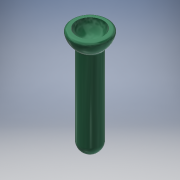
# Autodesk Inventor part: Component 4 (Pound)
Saved by Autodesk Inventor 2018 (Build 220112000, 112)
## iProperties
Created: 2023-03-14
Part Number: Component 4 (Pound)
Material: Generic
Document SubType Name: Modeling
Designer: Habib Mohamed
Density: 1 g/cm^3
Appearance: Olive Green
Author: Habib Mohamed
Autodesk Inventor part; units mm, degrees
ref_plane "YZ Plane" through (0, 0, 0) normal (1, 0, 0) x (0, 1, 0)
ref_plane "XZ Plane" through (0, 0, 0) normal (0, 1, 0) x (-1, 0, 0)
ref_plane "XY Plane" through (0, 0, 0) normal (0, 0, 1) x (1, 0, 0)
sketch "Sketch1" plane through (0, 0, 0) normal (1, 0, 0) x (0, 1, 0)
  line L0 (0, 0) -> (20, 0) construction
  arc A0 (20, 2.5) -> (17.5, 0) centre (20, 0) ccw
  arc A1 (19.4167, 3.451) -> (17.2678, 2.1875) centre (20, 0) ccw
  line L1 (2, 2) -> (16.8775, 2)
  line L2 (2, 2) -> (2, -2.5) construction
  arc A2 (2, 2) -> (0.0157, 0.25) centre (2, 0) ccw
  line L3 (0.25, 0) -> (0.0157, 0.25)
  line L4 (20, 0) -> (20, 2.958)
  line L5 (17.5, 0) -> (0.25, 0)
  arc A3 (20, 2.958) -> (19.4167, 3.451) centre (19.5, 2.958) ccw
  arc A4 (16.8775, 2) -> (17.2678, 2.1875) centre (16.8775, 2.5) ccw
  dimension "d0" = 20
  dimension "d1" = 5
  dimension "d2" = 7
  dimension "d3" = 2
  dimension "d4" = 2
  dimension "d5" = 0.25
  dimension "d6" = 0.25
  dimension "d7" = 1
  dimension "d8" = 1
  constraints: 12 end point, 10 point on circle, 5 centre point, 5 point on line, 4 tangent, 2 coincident, 1 collinear, 1 horizontal, 1 parallel, 1 perpendicular, 1 vertical
  measures "d0" distance of L0.start L0.end
  measures "d1" diameter of A0
  measures "d2" diameter of A1
  measures "d3" distance between parallel lines of L0 L1
  measures "d4" distance from line of L0.start L2
  measures "d5" distance of L3.start L0.start
  measures "d6" distance from line of L3.end L0
  measures "d7" diameter of A3
  measures "d8" diameter of A4
revolve "Revolution1" add sketch "Sketch1" angle 360 about axis through (0, 0, 0) along (0, 1, 0)
body "Solid1"
